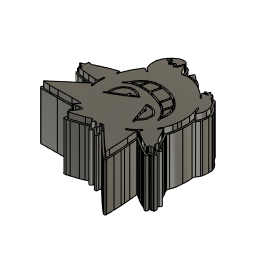
knop v2 (Autodesk Fusion 360 design; units mm, degrees)
Autodesk Fusion 360 part; units mm, degrees
(part 1 of 2)
sketch "Sketch5" plane through (0, 0, 0) normal (0, 0, 1) x (1, 0, 0)
  circle A0 centre (0, 52) radius 3.075
  circle A1 centre (0, 52) radius 12.5
  dimension "d73" = 6.15
  dimension "d74" = 25
  constraint concentric A0 A1
  measures "d73" diameter of A0
  measures "d74" diameter of A1
extrude "Extrude25" add sketch "Sketch5" along normal blind 14
sketch "Sketch6" plane through (0, 0, 0) normal (0, 0, -1) x (1, 0, 0)
  circle A0 centre (0, -52) radius 3.075
  circle A1 centre (0, -52) radius 12.5
  line L0 (0, -52) -> (0, -50.375)
  line L1 (0, -50.375) -> (-5.7654, -50.375)
  line L2 (0, -50.375) -> (4.6477, -50.375)
  dimension "d77" = 1.625
  constraint coincident A0.centre A1.centre
  constraint vertical L0
  constraint perpendicular L0 L1
  constraint perpendicular L0 L2
  measures "d77" distance of A0.centre L0.end
extrude "Extrude26" add sketch "Sketch6" against normal blind 14 contours A0 L1 L2 picked at (-0.148, -49.4191)
extrude "Extrude27" cut sketch "Sketch6" against normal blind 4 contours A0 L1 L2 picked at (-0.148, -49.4191)
sketch "Sketch7" plane through (0, 0, 14) normal (0, 0, 1) x (-1, 0, 0)
  arc A0 (-2.6106, -50.375) -> (2.6106, -50.375) centre (0, -52) ccw
  line L0 (-2.6106, -50.375) -> (2.6106, -50.375)
  circle A1 centre (0, -52) radius 12.5
extrude "Extrude28" add sketch "Sketch7" against normal blind 2 contours A0 L0
sketch "Sketch8" plane through (0, 0, 14) normal (0, 0, 1) x (-1, 0, 0)
  circle A0 centre (0, -52) radius 12.5
  spline S0 degree 3 poles (-7.7296, -35.2384) (-7.7669, -35.285) (-7.7902, -35.4107) (-7.7855, -35.555) knots 0 0 0 0 1 1 1 1
  spline S1 degree 3 poles (-7.7855, -35.555) (-7.7808, -35.6854) (-7.7576, -36.5886) (-7.7296, -37.5616) knots 0 0 0 0 1 1 1 1
  spline S2 degree 3 poles (-7.7296, -37.5616) (-7.7017, -38.5347) (-7.6691, -39.4053) (-7.6551, -39.4937) knots 0 0 0 0 1 1 1 1
  spline S3 degree 3 poles (-7.6551, -39.4937) (-7.6412, -39.5868) (-7.5993, -40.0245) (-7.562, -40.4714) knots 0 0 0 0 1 1 1 1
  spline S4 degree 3 poles (-7.562, -40.4714) (-7.427, -42.1521) (-7.278, -43.7118) (-7.2268, -44.0098) knots 0 0 0 0 1 1 1 1
  line L0 (-7.2268, -44.0098) -> (-7.1989, -44.1681)
  line L1 (-7.1989, -44.1681) -> (-7.3805, -44.0284)
  spline S5 degree 3 poles (-7.3805, -44.0284) (-7.6505, -43.8189) (-7.9857, -43.6001) (-8.2371, -43.4744) knots 0 0 0 0 1 1 1 1
  spline S6 degree 3 poles (-8.2371, -43.4744) (-8.3582, -43.4138) (-8.5164, -43.3114) (-8.5909, -43.2509) knots 0 0 0 0 1 1 1 1
  spline S7 degree 3 poles (-8.5909, -43.2509) (-8.6654, -43.1904) (-8.8191, -43.0926) (-8.9355, -43.0321) knots 0 0 0 0 1 1 1 1
  spline S8 degree 3 poles (-8.9355, -43.0321) (-9.0472, -42.9762) (-9.1962, -42.8877) (-9.2614, -42.8412) knots 0 0 0 0 1 1 1 1
  spline S9 degree 3 poles (-9.2614, -42.8412) (-9.3964, -42.7388) (-9.713, -42.5665) (-10.0063, -42.4268) knots 0 0 0 0 1 1 1 1
  spline S10 degree 3 poles (-10.0063, -42.4268) (-10.1227, -42.3756) (-10.2856, -42.2965) (-10.3694, -42.2546) knots 0 0 0 0 1 1 1 1
  spline S11 degree 3 poles (-10.3694, -42.2546) (-10.4579, -42.208) (-10.5556, -42.1708) (-10.5929, -42.1661) knots 0 0 0 0 1 1 1 1
  spline S12 degree 3 poles (-10.5929, -42.1661) (-10.6301, -42.1614) (-10.7279, -42.1149) (-10.8117, -42.059) knots 0 0 0 0 1 1 1 1
  spline S13 degree 3 poles (-10.8117, -42.059) (-10.8909, -42.0078) (-11.0398, -41.9194) (-11.1423, -41.8681) knots 0 0 0 0 1 1 1 1
  spline S14 degree 3 poles (-11.1423, -41.8681) (-11.24, -41.8123) (-11.403, -41.7052) (-11.5054, -41.6307) knots 0 0 0 0 1 1 1 1
  spline S15 degree 3 poles (-11.5054, -41.6307) (-11.7242, -41.4724) (-11.971, -41.4165) (-12.1246, -41.4864) knots 0 0 0 0 1 1 1 1
  spline S16 degree 3 poles (-12.1246, -41.4864) (-12.2689, -41.5515) (-12.3108, -41.7704) (-12.2457, -42.1242) knots 0 0 0 0 1 1 1 1
  spline S17 degree 3 poles (-12.2457, -42.1242) (-12.2177, -42.2732) (-12.1991, -42.4035) (-12.2084, -42.4082) knots 0 0 0 0 1 1 1 1
  spline S18 degree 3 poles (-12.2084, -42.4082) (-12.2177, -42.4175) (-12.2969, -42.4035) (-12.39, -42.3803) knots 0 0 0 0 1 1 1 1
  spline S19 degree 3 poles (-12.39, -42.3803) (-12.511, -42.343) (-12.6042, -42.3523) (-12.7531, -42.4035) knots 0 0 0 0 1 1 1 1
  spline S20 degree 3 poles (-12.7531, -42.4035) (-12.8602, -42.4408) (-13.0232, -42.4734) (-13.107, -42.4734) knots 0 0 0 0 1 1 1 1
  line L2 (-13.107, -42.4734) -> (-13.2653, -42.4734)
  line L3 (-13.2653, -42.4734) -> (-13.2653, -42.8924)
  line L4 (-13.2653, -42.8924) -> (-13.2653, -43.3067)
  line L5 (-13.2653, -43.3067) -> (-13.107, -43.4138)
  spline S21 degree 3 poles (-13.107, -43.4138) (-12.8975, -43.5582) (-12.5669, -43.8608) (-12.5669, -43.9073) knots 0 0 0 0 1 1 1 1
  spline S22 degree 3 poles (-12.5669, -43.9073) (-12.5669, -43.9306) (-12.6926, -44.0563) (-12.8462, -44.1913) knots 0 0 0 0 1 1 1 1
  spline S23 degree 3 poles (-12.8462, -44.1913) (-13.1302, -44.4381) (-13.2047, -44.5778) (-13.1489, -44.7547) knots 0 0 0 0 1 1 1 1
  spline S24 degree 3 poles (-13.1489, -44.7547) (-13.1209, -44.8478) (-12.9906, -44.9176) (-12.2503, -45.2482) knots 0 0 0 0 1 1 1 1
  spline S25 degree 3 poles (-12.2503, -45.2482) (-12.0827, -45.3227) (-11.9803, -45.4018) (-11.9244, -45.5042) knots 0 0 0 0 1 1 1 1
  spline S26 degree 3 poles (-11.9244, -45.5042) (-11.8825, -45.588) (-11.7894, -45.7231) (-11.7149, -45.8022) knots 0 0 0 0 1 1 1 1
  spline S27 degree 3 poles (-11.7149, -45.8022) (-11.6451, -45.886) (-11.5892, -45.9698) (-11.5892, -45.9838) knots 0 0 0 0 1 1 1 1
  spline S28 degree 3 poles (-11.5892, -45.9838) (-11.5892, -46.0024) (-11.4495, -46.3004) (-11.2819, -46.6542) knots 0 0 0 0 1 1 1 1
  spline S29 degree 3 poles (-11.2819, -46.6542) (-11.1143, -47.0034) (-10.956, -47.3339) (-10.9328, -47.3851) knots 0 0 0 0 1 1 1 1
  spline S30 degree 3 poles (-10.9328, -47.3851) (-10.9095, -47.4364) (-10.849, -47.5388) (-10.7977, -47.6179) knots 0 0 0 0 1 1 1 1
  spline S31 degree 3 poles (-10.7977, -47.6179) (-10.7465, -47.6924) (-10.6627, -47.8461) (-10.6115, -47.9531) knots 0 0 0 0 1 1 1 1
  spline S32 degree 3 poles (-10.6115, -47.9531) (-10.5556, -48.0602) (-10.4812, -48.158) (-10.4439, -48.172) knots 0 0 0 0 1 1 1 1
  spline S33 degree 3 poles (-10.4439, -48.172) (-10.4067, -48.1859) (-10.3787, -48.2278) (-10.3787, -48.2651) knots 0 0 0 0 1 1 1 1
  spline S34 degree 3 poles (-10.3787, -48.2651) (-10.3787, -48.3023) (-10.3135, -48.4466) (-10.2344, -48.5817) knots 0 0 0 0 1 1 1 1
  spline S35 degree 3 poles (-10.2344, -48.5817) (-10.1553, -48.7167) (-10.0808, -48.8657) (-10.0715, -48.9215) knots 0 0 0 0 1 1 1 1
  spline S36 degree 3 poles (-10.0715, -48.9215) (-10.0621, -48.9727) (-10.1366, -49.266) (-10.2391, -49.5733) knots 0 0 0 0 1 1 1 1
  spline S37 degree 3 poles (-10.2391, -49.5733) (-10.6208, -50.7373) (-10.6534, -50.9142) (-10.7698, -52.4878) knots 0 0 0 0 1 1 1 1
  spline S38 degree 3 poles (-10.7698, -52.4878) (-10.8396, -53.4515) (-10.8117, -54.7132) (-10.7093, -54.96) knots 0 0 0 0 1 1 1 1
  spline S39 degree 3 poles (-10.7093, -54.96) (-10.6348, -55.1509) (-10.6907, -55.3604) (-10.9141, -55.6956) knots 0 0 0 0 1 1 1 1
  spline S40 degree 3 poles (-10.9141, -55.6956) (-11.24, -56.1937) (-11.2819, -56.2682) (-11.389, -56.5336) knots 0 0 0 0 1 1 1 1
  spline S41 degree 3 poles (-11.389, -56.5336) (-11.5939, -57.0224) (-11.6544, -57.4228) (-11.6544, -58.3726) knots 0 0 0 0 1 1 1 1
  line L6 (-11.6544, -58.3726) -> (-11.6544, -59.2572)
  line L7 (-11.6544, -59.2572) -> (-11.4682, -59.6995)
  spline S42 degree 3 poles (-11.4682, -59.6995) (-11.3657, -59.9416) (-11.1795, -60.2814) (-11.0585, -60.4537) knots 0 0 0 0 1 1 1 1
  spline S43 degree 3 poles (-11.0585, -60.4537) (-10.8396, -60.7656) (-10.2251, -61.3755) (-10.132, -61.3755) knots 0 0 0 0 1 1 1 1
  spline S44 degree 3 poles (-10.132, -61.3755) (-10.104, -61.3755) (-9.969, -61.4407) (-9.834, -61.5245) knots 0 0 0 0 1 1 1 1
  spline S45 degree 3 poles (-9.834, -61.5245) (-9.6478, -61.6363) (-9.5733, -61.7154) (-9.536, -61.8411) knots 0 0 0 0 1 1 1 1
  spline S46 degree 3 poles (-9.536, -61.8411) (-9.5081, -61.9296) (-9.401, -62.1251) (-9.3033, -62.2787) knots 0 0 0 0 1 1 1 1
  spline S47 degree 3 poles (-9.3033, -62.2787) (-9.2008, -62.4277) (-9.1217, -62.5674) (-9.1217, -62.586) knots 0 0 0 0 1 1 1 1
  spline S48 degree 3 poles (-9.1217, -62.586) (-9.1217, -62.6046) (-9.0193, -62.7164) (-8.8889, -62.8374) knots 0 0 0 0 1 1 1 1
  spline S49 degree 3 poles (-8.8889, -62.8374) (-8.6096, -63.0981) (-8.4606, -63.1168) (-8.3349, -62.9073) knots 0 0 0 0 1 1 1 1
  line L8 (-8.3349, -62.9073) -> (-8.2418, -62.7583)
  line L9 (-8.2418, -62.7583) -> (-8.144, -62.9724)
  spline S50 degree 3 poles (-8.144, -62.9724) (-8.0648, -63.1447) (-8.0043, -63.2006) (-7.8181, -63.2797) knots 0 0 0 0 1 1 1 1
  spline S51 degree 3 poles (-7.8181, -63.2797) (-7.4084, -63.4566) (-7.3292, -63.4101) (-7.2548, -62.9538) knots 0 0 0 0 1 1 1 1
  spline S52 degree 3 poles (-7.2548, -62.9538) (-7.2268, -62.7909) (-7.1989, -62.6512) (-7.1942, -62.6465) knots 0 0 0 0 1 1 1 1
  spline S53 degree 3 poles (-7.1942, -62.6465) (-7.1849, -62.6372) (-7.0871, -62.6838) (-6.9754, -62.749) knots 0 0 0 0 1 1 1 1
  spline S54 degree 3 poles (-6.9754, -62.749) (-6.8637, -62.8095) (-6.7147, -62.8654) (-6.6449, -62.8654) knots 0 0 0 0 1 1 1 1
  spline S55 degree 3 poles (-6.6449, -62.8654) (-6.3981, -62.8654) (-6.3003, -62.5395) (-6.4447, -62.1996) knots 0 0 0 0 1 1 1 1
  spline S56 degree 3 poles (-6.4447, -62.1996) (-6.5238, -62.0041) (-6.5378, -61.748) (-6.4633, -61.748) knots 0 0 0 0 1 1 1 1
  spline S57 degree 3 poles (-6.4633, -61.748) (-6.4353, -61.748) (-6.3562, -61.8085) (-6.2864, -61.8783) knots 0 0 0 0 1 1 1 1
  spline S58 degree 3 poles (-6.2864, -61.8783) (-6.1141, -62.046) (-5.467, -62.4789) (-5.0247, -62.7164) knots 0 0 0 0 1 1 1 1
  spline S59 degree 3 poles (-5.0247, -62.7164) (-4.5032, -62.9957) (-4.4194, -63.033) (-4.1261, -63.1633) knots 0 0 0 0 1 1 1 1
  spline S60 degree 3 poles (-4.1261, -63.1633) (-3.9352, -63.2518) (-3.8282, -63.3309) (-3.763, -63.4473) knots 0 0 0 0 1 1 1 1
  spline S61 degree 3 poles (-3.763, -63.4473) (-3.7071, -63.5358) (-3.6512, -63.6103) (-3.6326, -63.6103) knots 0 0 0 0 1 1 1 1
  spline S62 degree 3 poles (-3.6326, -63.6103) (-3.614, -63.6103) (-3.5674, -63.6661) (-3.5302, -63.736) knots 0 0 0 0 1 1 1 1
  spline S63 degree 3 poles (-3.5302, -63.736) (-3.4929, -63.8058) (-3.3719, -63.9455) (-3.2648, -64.0479) knots 0 0 0 0 1 1 1 1
  spline S64 degree 3 poles (-3.2648, -64.0479) (-3.1531, -64.155) (-2.9762, -64.3226) (-2.8691, -64.4297) knots 0 0 0 0 1 1 1 1
  spline S65 degree 3 poles (-2.8691, -64.4297) (-2.2918, -64.9884) (-1.4631, -65.3143) (-1.2442, -65.0628) knots 0 0 0 0 1 1 1 1
  spline S66 degree 3 poles (-1.2442, -65.0628) (-1.2023, -65.0209) (-1.0953, -64.7835) (-0.9975, -64.5414) knots 0 0 0 0 1 1 1 1
  spline S67 degree 3 poles (-0.9975, -64.5414) (-0.6716, -63.7127) (-0.6157, -63.6429) (-0.2014, -63.5916) knots 0 0 0 0 1 1 1 1
  spline S68 degree 3 poles (-0.2014, -63.5916) (0.0314, -63.5637) (0.0407, -63.5637) (0.1851, -63.736) knots 0 0 0 0 1 1 1 1
  spline S69 degree 3 poles (0.1851, -63.736) (0.2642, -63.8337) (0.3899, -63.9734) (0.4644, -64.0526) knots 0 0 0 0 1 1 1 1
  spline S70 degree 3 poles (0.4644, -64.0526) (0.5901, -64.1783) (1.1302, -65.2724) (1.2885, -65.724) knots 0 0 0 0 1 1 1 1
  spline S71 degree 3 poles (1.2885, -65.724) (1.4654, -66.2175) (1.7866, -66.5853) (2.1405, -66.711) knots 0 0 0 0 1 1 1 1
  spline S72 degree 3 poles (2.1405, -66.711) (2.2475, -66.7482) (2.6107, -66.7715) (3.1368, -66.7761) knots 0 0 0 0 1 1 1 1
  spline S73 degree 3 poles (3.1368, -66.7761) (3.9562, -66.7808) (3.9655, -66.7761) (4.1843, -66.6504) knots 0 0 0 0 1 1 1 1
  spline S74 degree 3 poles (4.1843, -66.6504) (4.3054, -66.5806) (4.4264, -66.5015) (4.4543, -66.4735) knots 0 0 0 0 1 1 1 1
  spline S75 degree 3 poles (4.4543, -66.4735) (4.4823, -66.4502) (4.6313, -66.3432) (4.7802, -66.2407) knots 0 0 0 0 1 1 1 1
  spline S76 degree 3 poles (4.7802, -66.2407) (5.3529, -65.8497) (6.1863, -64.872) (6.5029, -64.2155) knots 0 0 0 0 1 1 1 1
  spline S77 degree 3 poles (6.5029, -64.2155) (6.596, -64.0246) (6.6891, -63.8291) (6.7077, -63.7872) knots 0 0 0 0 1 1 1 1
  spline S78 degree 3 poles (6.7077, -63.7872) (6.866, -63.4892) (7.0615, -62.2089) (7.0196, -61.7806) knots 0 0 0 0 1 1 1 1
  spline S79 degree 3 poles (7.0196, -61.7806) (6.9498, -61.0962) (6.8753, -60.6725) (6.7729, -60.4258) knots 0 0 0 0 1 1 1 1
  spline S80 degree 3 poles (6.7729, -60.4258) (6.6332, -60.0812) (6.6332, -60.0673) (6.7775, -59.9323) knots 0 0 0 0 1 1 1 1
  spline S81 degree 3 poles (6.7775, -59.9323) (6.8427, -59.8717) (6.8939, -59.7972) (6.8939, -59.7647) knots 0 0 0 0 1 1 1 1
  spline S82 degree 3 poles (6.8939, -59.7647) (6.8939, -59.7321) (6.9219, -59.6762) (6.9591, -59.639) knots 0 0 0 0 1 1 1 1
  spline S83 degree 3 poles (6.9591, -59.639) (7.1593, -59.4434) (8.4303, -57.1575) (8.4303, -57.0038) knots 0 0 0 0 1 1 1 1
  spline S84 degree 3 poles (8.4303, -57.0038) (8.4303, -56.9759) (8.4955, -56.8316) (8.57, -56.6872) knots 0 0 0 0 1 1 1 1
  spline S85 degree 3 poles (8.57, -56.6872) (8.6491, -56.5429) (8.7097, -56.4032) (8.7097, -56.3707) knots 0 0 0 0 1 1 1 1
  spline S86 degree 3 poles (8.7097, -56.3707) (8.7097, -56.2636) (8.8726, -56.1705) (9.2683, -56.0494) knots 0 0 0 0 1 1 1 1
  spline S87 degree 3 poles (9.2683, -56.0494) (10.1064, -55.798) (10.5161, -55.6537) (10.7489, -55.5373) knots 0 0 0 0 1 1 1 1
  spline S88 degree 3 poles (10.7489, -55.5373) (10.8792, -55.4721) (11.0328, -55.4162) (11.0841, -55.4162) knots 0 0 0 0 1 1 1 1
  spline S89 degree 3 poles (11.0841, -55.4162) (11.1353, -55.4162) (11.3913, -55.3138) (11.6567, -55.1881) knots 0 0 0 0 1 1 1 1
  spline S90 degree 3 poles (11.6567, -55.1881) (11.9174, -55.0624) (12.1828, -54.946) (12.248, -54.9274) knots 0 0 0 0 1 1 1 1
  spline S91 degree 3 poles (12.248, -54.9274) (12.3132, -54.9088) (12.4482, -54.8436) (12.5506, -54.7877) knots 0 0 0 0 1 1 1 1
  spline S92 degree 3 poles (12.5506, -54.7877) (12.653, -54.7272) (12.8486, -54.648) (12.9789, -54.6015) knots 0 0 0 0 1 1 1 1
  spline S93 degree 3 poles (12.9789, -54.6015) (13.1139, -54.5596) (13.235, -54.5084) (13.249, -54.4851) knots 0 0 0 0 1 1 1 1
  spline S94 degree 3 poles (13.249, -54.4851) (13.2955, -54.4106) (14.2639, -53.9683) (14.3384, -53.9869) knots 0 0 0 0 1 1 1 1
  spline S95 degree 3 poles (14.3384, -53.9869) (14.3803, -54.0009) (14.5619, -54.0614) (14.7388, -54.1266) knots 0 0 0 0 1 1 1 1
  spline S96 degree 3 poles (14.7388, -54.1266) (15.0833, -54.2523) (15.2882, -54.2477) (15.3487, -54.1173) knots 0 0 0 0 1 1 1 1
  spline S97 degree 3 poles (15.3487, -54.1173) (15.372, -54.0754) (15.3999, -53.8333) (15.4139, -53.5772) knots 0 0 0 0 1 1 1 1
  line L10 (15.4139, -53.5772) -> (15.4371, -53.1117)
  line L11 (15.4371, -53.1117) -> (15.7863, -52.9953)
  spline S98 degree 3 poles (15.7863, -52.9953) (16.3869, -52.7951) (16.6756, -52.5716) (16.6057, -52.3621) knots 0 0 0 0 1 1 1 1
  spline S99 degree 3 poles (16.6057, -52.3621) (16.5731, -52.2597) (16.0796, -51.9291) (15.8329, -51.8407) knots 0 0 0 0 1 1 1 1
  spline S100 degree 3 poles (15.8329, -51.8407) (15.7444, -51.8081) (15.6373, -51.7708) (15.6001, -51.7569) knots 0 0 0 0 1 1 1 1
  spline S101 degree 3 poles (15.6001, -51.7569) (15.5535, -51.7382) (15.6001, -51.6917) (15.7491, -51.6172) knots 0 0 0 0 1 1 1 1
  spline S102 degree 3 poles (15.7491, -51.6172) (15.9353, -51.5241) (15.9726, -51.4822) (15.9726, -51.3704) knots 0 0 0 0 1 1 1 1
  spline S103 degree 3 poles (15.9726, -51.3704) (15.9726, -51.147) (15.8143, -51.0632) (14.9809, -50.849) knots 0 0 0 0 1 1 1 1
  spline S104 degree 3 poles (14.9809, -50.849) (14.7202, -50.7838) (13.7937, -50.6674) (13.519, -50.6674) knots 0 0 0 0 1 1 1 1
  spline S105 degree 3 poles (13.519, -50.6674) (13.3886, -50.6674) (13.2629, -50.6441) (13.249, -50.6209) knots 0 0 0 0 1 1 1 1
  spline S106 degree 3 poles (13.249, -50.6209) (13.235, -50.5929) (13.0162, -50.5743) (12.7555, -50.5743) knots 0 0 0 0 1 1 1 1
  spline S107 degree 3 poles (12.7555, -50.5743) (12.4994, -50.5743) (12.1363, -50.5417) (11.9454, -50.5045) knots 0 0 0 0 1 1 1 1
  spline S108 degree 3 poles (11.9454, -50.5045) (11.7545, -50.4626) (11.3215, -50.4114) (10.9816, -50.3881) knots 0 0 0 0 1 1 1 1
  spline S109 degree 3 poles (10.9816, -50.3881) (10.2786, -50.3369) (9.8829, -50.2763) (9.8084, -50.2018) knots 0 0 0 0 1 1 1 1
  spline S110 degree 3 poles (9.8084, -50.2018) (9.7572, -50.146) (9.962, -49.9411) (10.5906, -49.4104) knots 0 0 0 0 1 1 1 1
  spline S111 degree 3 poles (10.5906, -49.4104) (10.7582, -49.2707) (11.0282, -49.0333) (11.1865, -48.8843) knots 0 0 0 0 1 1 1 1
  spline S112 degree 3 poles (11.1865, -48.8843) (11.3448, -48.74) (11.4891, -48.6189) (11.5031, -48.6189) knots 0 0 0 0 1 1 1 1
  spline S113 degree 3 poles (11.5031, -48.6189) (11.5217, -48.6189) (11.6055, -48.5537) (11.694, -48.4792) knots 0 0 0 0 1 1 1 1
  spline S114 degree 3 poles (11.694, -48.4792) (11.7824, -48.4001) (11.9267, -48.2744) (12.0152, -48.1999) knots 0 0 0 0 1 1 1 1
  spline S115 degree 3 poles (12.0152, -48.1999) (12.1037, -48.1207) (12.3364, -47.9206) (12.5273, -47.7529) knots 0 0 0 0 1 1 1 1
  spline S116 degree 3 poles (12.5273, -47.7529) (12.7182, -47.5807) (12.937, -47.3991) (13.0208, -47.3432) knots 0 0 0 0 1 1 1 1
  spline S117 degree 3 poles (13.0208, -47.3432) (13.1745, -47.2408) (14.2127, -46.3749) (14.4594, -46.1374) knots 0 0 0 0 1 1 1 1
  spline S118 degree 3 poles (14.4594, -46.1374) (14.5386, -46.0676) (14.6643, -45.9465) (14.7388, -45.8767) knots 0 0 0 0 1 1 1 1
  spline S119 degree 3 poles (14.7388, -45.8767) (14.8179, -45.8022) (15.1531, -45.5089) (15.4837, -45.2202) knots 0 0 0 0 1 1 1 1
  spline S120 degree 3 poles (15.4837, -45.2202) (15.8189, -44.9362) (16.1774, -44.6197) (16.2845, -44.5219) knots 0 0 0 0 1 1 1 1
  spline S121 degree 3 poles (16.2845, -44.5219) (16.3916, -44.4241) (16.5685, -44.2798) (16.6802, -44.2053) knots 0 0 0 0 1 1 1 1
  spline S122 degree 3 poles (16.6802, -44.2053) (16.792, -44.1308) (16.9177, -44.0284) (16.9596, -43.9772) knots 0 0 0 0 1 1 1 1
  spline S123 degree 3 poles (16.9596, -43.9772) (17.0992, -43.8235) (17.2808, -43.4464) (17.2529, -43.3626) knots 0 0 0 0 1 1 1 1
  spline S124 degree 3 poles (17.2529, -43.3626) (17.2389, -43.3207) (17.1504, -43.2369) (17.0573, -43.1717) knots 0 0 0 0 1 1 1 1
  line L12 (17.0573, -43.1717) -> (16.8851, -43.0553)
  line L13 (16.8851, -43.0553) -> (12.5785, -43.06)
  spline S125 degree 3 poles (12.5785, -43.06) (9.0262, -43.0693) (8.1975, -43.0786) (7.8623, -43.1391) knots 0 0 0 0 1 1 1 1
  spline S126 degree 3 poles (7.8623, -43.1391) (7.4666, -43.2043) (7.3409, -43.1764) (7.5597, -43.074) knots 0 0 0 0 1 1 1 1
  spline S127 degree 3 poles (7.5597, -43.074) (7.6156, -43.046) (7.7133, -42.9529) (7.7785, -42.8691) knots 0 0 0 0 1 1 1 1
  spline S128 degree 3 poles (7.7785, -42.8691) (7.8437, -42.7853) (7.9927, -42.5851) (8.1184, -42.4268) knots 0 0 0 0 1 1 1 1
  spline S129 degree 3 poles (8.1184, -42.4268) (8.3512, -42.1195) (8.3977, -41.9287) (8.2627, -41.8169) knots 0 0 0 0 1 1 1 1
  spline S130 degree 3 poles (8.2627, -41.8169) (8.2022, -41.7657) (8.0951, -41.7704) (7.6249, -41.8355) knots 0 0 0 0 1 1 1 1
  spline S131 degree 3 poles (7.6249, -41.8355) (7.3129, -41.8821) (6.9545, -41.9147) (6.8241, -41.9147) knots 0 0 0 0 1 1 1 1
  spline S132 degree 3 poles (6.8241, -41.9147) (6.6984, -41.9147) (6.4284, -41.9566) (6.2282, -42.0032) knots 0 0 0 0 1 1 1 1
  line L14 (6.2282, -42.0032) -> (5.865, -42.087)
  line L15 (5.865, -42.087) -> (5.9395, -41.9892)
  spline S133 degree 3 poles (5.9395, -41.9892) (5.9814, -41.938) (6.0559, -41.803) (6.1071, -41.6959) knots 0 0 0 0 1 1 1 1
  spline S134 degree 3 poles (6.1071, -41.6959) (6.1583, -41.5888) (6.2142, -41.4864) (6.2375, -41.4771) knots 0 0 0 0 1 1 1 1
  spline S135 degree 3 poles (6.2375, -41.4771) (6.3027, -41.4352) (6.6611, -40.8113) (6.9731, -40.1967) knots 0 0 0 0 1 1 1 1
  spline S136 degree 3 poles (6.9731, -40.1967) (7.3502, -39.4518) (7.3595, -39.2749) (7.0103, -39.2423) knots 0 0 0 0 1 1 1 1
  spline S137 degree 3 poles (7.0103, -39.2423) (6.9079, -39.233) (6.6891, -39.2656) (6.5215, -39.3122) knots 0 0 0 0 1 1 1 1
  spline S138 degree 3 poles (6.5215, -39.3122) (6.3539, -39.3634) (6, -39.4611) (5.73, -39.5356) knots 0 0 0 0 1 1 1 1
  spline S139 degree 3 poles (5.73, -39.5356) (4.8501, -39.7824) (3.2485, -40.3318) (2.8202, -40.5413) knots 0 0 0 0 1 1 1 1
  spline S140 degree 3 poles (2.8202, -40.5413) (2.2382, -40.8253) (1.9542, -40.9417) (1.9123, -40.9137) knots 0 0 0 0 1 1 1 1
  spline S141 degree 3 poles (1.9123, -40.9137) (1.889, -40.8998) (1.8146, -40.774) (1.7494, -40.6297) knots 0 0 0 0 1 1 1 1
  spline S142 degree 3 poles (1.7494, -40.6297) (1.6842, -40.49) (1.5538, -40.2899) (1.4607, -40.1874) knots 0 0 0 0 1 1 1 1
  spline S143 degree 3 poles (1.4607, -40.1874) (1.1767, -39.8755) (0.9858, -39.95) (0.7018, -40.504) knots 0 0 0 0 1 1 1 1
  spline S144 degree 3 poles (0.7018, -40.504) (0.646, -40.6158) (0.5901, -40.7042) (0.5761, -40.7042) knots 0 0 0 0 1 1 1 1
  spline S145 degree 3 poles (0.5761, -40.7042) (0.5668, -40.7042) (0.4877, -40.6344) (0.4039, -40.5506) knots 0 0 0 0 1 1 1 1
  spline S146 degree 3 poles (0.4039, -40.5506) (0.3201, -40.4714) (0.1199, -40.2759) (-0.0477, -40.1176) knots 0 0 0 0 1 1 1 1
  spline S147 degree 3 poles (-0.0477, -40.1176) (-0.2107, -39.964) (-0.4341, -39.7405) (-0.5412, -39.6194) knots 0 0 0 0 1 1 1 1
  spline S148 degree 3 poles (-0.5412, -39.6194) (-0.6483, -39.503) (-0.7833, -39.4006) (-0.8438, -39.3913) knots 0 0 0 0 1 1 1 1
  spline S149 degree 3 poles (-0.8438, -39.3913) (-1.0534, -39.3634) (-1.1139, -39.4844) (-1.1884, -40.1036) knots 0 0 0 0 1 1 1 1
  spline S150 degree 3 poles (-1.1884, -40.1036) (-1.2722, -40.802) (-1.2861, -40.8579) (-1.3606, -40.7182) knots 0 0 0 0 1 1 1 1
  spline S151 degree 3 poles (-1.3606, -40.7182) (-1.3932, -40.6623) (-1.5422, -40.5087) (-1.6912, -40.369) knots 0 0 0 0 1 1 1 1
  spline S152 degree 3 poles (-1.6912, -40.369) (-1.8448, -40.234) (-2.0124, -40.071) (-2.0636, -40.0105) knots 0 0 0 0 1 1 1 1
  spline S153 degree 3 poles (-2.0636, -40.0105) (-2.1195, -39.9453) (-2.194, -39.8615) (-2.2406, -39.8243) knots 0 0 0 0 1 1 1 1
  spline S154 degree 3 poles (-2.2406, -39.8243) (-2.2825, -39.7824) (-2.5339, -39.5403) (-2.7992, -39.2842) knots 0 0 0 0 1 1 1 1
  spline S155 degree 3 poles (-2.7992, -39.2842) (-3.3766, -38.7255) (-4.2658, -37.8968) (-5.0945, -37.1333) knots 0 0 0 0 1 1 1 1
  spline S156 degree 3 poles (-5.0945, -37.1333) (-5.4251, -36.8307) (-5.7789, -36.5048) (-5.872, -36.4163) knots 0 0 0 0 1 1 1 1
  spline S157 degree 3 poles (-5.872, -36.4163) (-6.1746, -36.137) (-6.4726, -35.8902) (-6.6774, -35.7459) knots 0 0 0 0 1 1 1 1
  spline S158 degree 3 poles (-6.6774, -35.7459) (-6.7845, -35.6667) (-7.008, -35.5084) (-7.1663, -35.3827) knots 0 0 0 0 1 1 1 1
  spline S159 degree 3 poles (-7.1663, -35.3827) (-7.4689, -35.1546) (-7.6226, -35.1127) (-7.7296, -35.2384) knots 0 0 0 0 1 1 1 1
  spline S160 degree 3 poles (-7.3153, -35.6807) (-7.3479, -35.6993) (-7.3618, -35.7273) (-7.3525, -35.7366) knots 0 0 0 0 1 1 1 1
  spline S161 degree 3 poles (-7.3525, -35.7366) (-7.3386, -35.7459) (-7.1523, -35.8995) (-6.9335, -36.0764) knots 0 0 0 0 1 1 1 1
  spline S162 degree 3 poles (-6.9335, -36.0764) (-6.5704, -36.3698) (-5.5275, -37.2962) (-5.4204, -37.4173) knots 0 0 0 0 1 1 1 1
  spline S163 degree 3 poles (-5.4204, -37.4173) (-5.3925, -37.4499) (-4.9735, -37.8363) (-4.4893, -38.2832) knots 0 0 0 0 1 1 1 1
  spline S164 degree 3 poles (-4.4893, -38.2832) (-3.6, -39.098) (-2.9715, -39.6939) (-2.4454, -40.22) knots 0 0 0 0 1 1 1 1
  spline S165 degree 3 poles (-2.4454, -40.22) (-2.2871, -40.3783) (-2.0031, -40.6483) (-1.8122, -40.8206) knots 0 0 0 0 1 1 1 1
  spline S166 degree 3 poles (-1.8122, -40.8206) (-1.6214, -40.9929) (-1.3979, -41.1931) (-1.3187, -41.2629) knots 0 0 0 0 1 1 1 1
  spline S167 degree 3 poles (-1.3187, -41.2629) (-1.0813, -41.4724) (-0.9835, -41.5096) (-0.7135, -41.4771) knots 0 0 0 0 1 1 1 1
  spline S168 degree 3 poles (-0.7135, -41.4771) (-0.369, -41.4352) (-0.2293, -41.3746) (-0.2293, -41.2629) knots 0 0 0 0 1 1 1 1
  spline S169 degree 3 poles (-0.2293, -41.2629) (-0.2293, -41.1465) (-0.3969, -41.0999) (-0.6809, -41.1418) knots 0 0 0 0 1 1 1 1
  line L16 (-0.6809, -41.1418) -> (-0.8951, -41.1698)
  line L17 (-0.8951, -41.1698) -> (-0.8671, -40.6949)
  spline S170 degree 3 poles (-0.8671, -40.6949) (-0.8392, -40.2014) (-0.8066, -40.0384) (-0.7368, -40.0617) knots 0 0 0 0 1 1 1 1
  spline S171 degree 3 poles (-0.7368, -40.0617) (-0.7181, -40.071) (-0.504, -40.2666) (-0.2665, -40.4994) knots 0 0 0 0 1 1 1 1
  spline S172 degree 3 poles (-0.2665, -40.4994) (0.4132, -41.1605) (0.8555, -41.4445) (0.9067, -41.2489) knots 0 0 0 0 1 1 1 1
  spline S173 degree 3 poles (0.9067, -41.2489) (0.9719, -40.9929) (1.1488, -40.518) (1.1767, -40.518) knots 0 0 0 0 1 1 1 1
  spline S174 degree 3 poles (1.1767, -40.518) (1.1953, -40.518) (1.2978, -40.6902) (1.4049, -40.8998) knots 0 0 0 0 1 1 1 1
  spline S175 degree 3 poles (1.4049, -40.8998) (1.647, -41.3933) (1.6656, -41.4165) (1.8378, -41.3886) knots 0 0 0 0 1 1 1 1
  spline S176 degree 3 poles (1.8378, -41.3886) (1.9868, -41.3653) (2.7178, -41.0767) (3.053, -40.9044) knots 0 0 0 0 1 1 1 1
  spline S177 degree 3 poles (3.053, -40.9044) (3.3696, -40.7461) (5.1667, -40.1548) (6.3818, -39.815) knots 0 0 0 0 1 1 1 1
  spline S178 degree 3 poles (6.3818, -39.815) (6.7589, -39.7079) (6.7868, -39.7079) (6.6984, -39.8057) knots 0 0 0 0 1 1 1 1
  spline S179 degree 3 poles (6.6984, -39.8057) (6.6565, -39.8522) (6.6099, -39.936) (6.596, -39.9919) knots 0 0 0 0 1 1 1 1
  spline S180 degree 3 poles (6.596, -39.9919) (6.5634, -40.0897) (5.9861, -41.0906) (5.6695, -41.5888) knots 0 0 0 0 1 1 1 1
  spline S181 degree 3 poles (5.6695, -41.5888) (5.4786, -41.8914) (5.2831, -42.3663) (5.325, -42.4129) knots 0 0 0 0 1 1 1 1
  spline S182 degree 3 poles (5.325, -42.4129) (5.3855, -42.4734) (5.8883, -42.4827) (6.2654, -42.4268) knots 0 0 0 0 1 1 1 1
  spline S183 degree 3 poles (6.2654, -42.4268) (6.4703, -42.3989) (6.8055, -42.357) (7.0103, -42.3337) knots 0 0 0 0 1 1 1 1
  spline S184 degree 3 poles (7.0103, -42.3337) (7.2152, -42.3104) (7.4666, -42.2778) (7.569, -42.2639) knots 0 0 0 0 1 1 1 1
  line L18 (7.569, -42.2639) -> (7.7552, -42.2359)
  line L19 (7.7552, -42.2359) -> (7.6342, -42.343)
  spline S185 degree 3 poles (7.6342, -42.343) (7.5085, -42.4548) (7.1267, -42.9576) (7.1267, -43.0134) knots 0 0 0 0 1 1 1 1
  spline S186 degree 3 poles (7.1267, -43.0134) (7.1267, -43.0833) (6.9684, -43.2183) (6.8846, -43.2183) knots 0 0 0 0 1 1 1 1
  spline S187 degree 3 poles (6.8846, -43.2183) (6.7682, -43.2183) (6.7263, -43.3487) (6.8101, -43.4371) knots 0 0 0 0 1 1 1 1
  spline S188 degree 3 poles (6.8101, -43.4371) (6.8707, -43.4976) (7.1919, -43.5069) (9.1985, -43.5069) knots 0 0 0 0 1 1 1 1
  spline S189 degree 3 poles (9.1985, -43.5069) (10.4695, -43.5069) (12.0757, -43.479) (12.7648, -43.4464) knots 0 0 0 0 1 1 1 1
  spline S190 degree 3 poles (12.7648, -43.4464) (13.4585, -43.4185) (14.4362, -43.4045) (14.939, -43.4185) knots 0 0 0 0 1 1 1 1
  spline S191 degree 3 poles (14.939, -43.4185) (15.8422, -43.4418) (16.7175, -43.5302) (16.7175, -43.6001) knots 0 0 0 0 1 1 1 1
  spline S192 degree 3 poles (16.7175, -43.6001) (16.7175, -43.6187) (16.6616, -43.6699) (16.5918, -43.7165) knots 0 0 0 0 1 1 1 1
  spline S193 degree 3 poles (16.5918, -43.7165) (16.5173, -43.7584) (16.3916, -43.8654) (16.3078, -43.9492) knots 0 0 0 0 1 1 1 1
  spline S194 degree 3 poles (16.3078, -43.9492) (16.224, -44.033) (16.0051, -44.2239) (15.8189, -44.3682) knots 0 0 0 0 1 1 1 1
  spline S195 degree 3 poles (15.8189, -44.3682) (15.3906, -44.7128) (14.3431, -45.6299) (13.8309, -46.1048) knots 0 0 0 0 1 1 1 1
  spline S196 degree 3 poles (13.8309, -46.1048) (13.6121, -46.3097) (13.235, -46.6263) (12.9929, -46.8125) knots 0 0 0 0 1 1 1 1
  spline S197 degree 3 poles (12.9929, -46.8125) (12.7508, -46.9941) (12.2945, -47.3665) (11.9826, -47.6366) knots 0 0 0 0 1 1 1 1
  spline S198 degree 3 poles (11.9826, -47.6366) (11.666, -47.9066) (11.2424, -48.2651) (11.0328, -48.4327) knots 0 0 0 0 1 1 1 1
  spline S199 degree 3 poles (11.0328, -48.4327) (10.828, -48.6003) (10.5347, -48.8517) (10.3904, -48.9914) knots 0 0 0 0 1 1 1 1
  spline S200 degree 3 poles (10.3904, -48.9914) (9.9434, -49.415) (9.7293, -49.6059) (9.7153, -49.5919) knots 0 0 0 0 1 1 1 1
  spline S201 degree 3 poles (9.7153, -49.5919) (9.706, -49.5826) (9.6734, -49.4383) (9.6455, -49.2754) knots 0 0 0 0 1 1 1 1
  spline S202 degree 3 poles (9.6455, -49.2754) (9.557, -48.8144) (9.5197, -48.7493) (9.3708, -48.7679) knots 0 0 0 0 1 1 1 1
  spline S203 degree 3 poles (9.3708, -48.7679) (9.259, -48.7819) (9.2451, -48.8005) (9.2497, -48.9448) knots 0 0 0 0 1 1 1 1
  spline S204 degree 3 poles (9.2497, -48.9448) (9.2497, -49.0333) (9.2916, -49.2754) (9.3382, -49.4802) knots 0 0 0 0 1 1 1 1
  spline S205 degree 3 poles (9.3382, -49.4802) (9.4173, -49.8434) (9.4313, -50.3136) (9.3894, -52.0408) knots 0 0 0 0 1 1 1 1
  spline S206 degree 3 poles (9.3894, -52.0408) (9.3847, -52.2923) (9.394, -52.3202) (9.4825, -52.3342) knots 0 0 0 0 1 1 1 1
  spline S207 degree 3 poles (9.4825, -52.3342) (9.6268, -52.3528) (9.6455, -52.2643) (9.6874, -51.4682) knots 0 0 0 0 1 1 1 1
  spline S208 degree 3 poles (9.6874, -51.4682) (9.706, -51.0771) (9.7339, -50.7466) (9.7525, -50.7279) knots 0 0 0 0 1 1 1 1
  spline S209 degree 3 poles (9.7525, -50.7279) (9.7665, -50.7093) (10.0691, -50.7233) (10.423, -50.7512) knots 0 0 0 0 1 1 1 1
  spline S210 degree 3 poles (10.423, -50.7512) (10.7721, -50.7792) (11.5729, -50.849) (12.2014, -50.9002) knots 0 0 0 0 1 1 1 1
  spline S211 degree 3 poles (12.2014, -50.9002) (12.83, -50.9514) (13.5423, -51.0212) (13.7844, -51.0585) knots 0 0 0 0 1 1 1 1
  spline S212 degree 3 poles (13.7844, -51.0585) (14.9855, -51.2447) (15.209, -51.2866) (15.2928, -51.3285) knots 0 0 0 0 1 1 1 1
  spline S213 degree 3 poles (15.2928, -51.3285) (15.372, -51.3704) (15.372, -51.3797) (15.3068, -51.4496) knots 0 0 0 0 1 1 1 1
  spline S214 degree 3 poles (15.3068, -51.4496) (15.2416, -51.5101) (15.209, -51.5148) (15.0461, -51.4589) knots 0 0 0 0 1 1 1 1
  spline S215 degree 3 poles (15.0461, -51.4589) (14.9436, -51.4263) (14.8272, -51.4123) (14.79, -51.4263) knots 0 0 0 0 1 1 1 1
  spline S216 degree 3 poles (14.79, -51.4263) (14.7015, -51.4589) (14.6969, -51.5939) (14.776, -51.6917) knots 0 0 0 0 1 1 1 1
  spline S217 degree 3 poles (14.776, -51.6917) (14.8598, -51.7988) (15.4744, -52.1572) (15.5815, -52.1572) knots 0 0 0 0 1 1 1 1
  spline S218 degree 3 poles (15.5815, -52.1572) (15.628, -52.1619) (15.763, -52.2131) (15.8794, -52.2736) knots 0 0 0 0 1 1 1 1
  line L20 (15.8794, -52.2736) -> (16.0889, -52.3807)
  line L21 (16.0889, -52.3807) -> (15.9027, -52.4599)
  spline S219 degree 3 poles (15.9027, -52.4599) (15.0181, -52.8277) (14.9949, -52.8509) (14.9949, -53.3957) knots 0 0 0 0 1 1 1 1
  line L22 (14.9949, -53.3957) -> (14.9949, -53.7821)
  line L23 (14.9949, -53.7821) -> (14.7062, -53.661)
  spline S220 degree 3 poles (14.7062, -53.661) (14.3617, -53.5214) (14.1754, -53.5353) (13.7611, -53.7355) knots 0 0 0 0 1 1 1 1
  spline S221 degree 3 poles (13.7611, -53.7355) (13.6075, -53.81) (13.2629, -53.973) (12.9929, -54.094) knots 0 0 0 0 1 1 1 1
  spline S222 degree 3 poles (12.9929, -54.094) (12.7229, -54.2151) (12.234, -54.4339) (11.8988, -54.5875) knots 0 0 0 0 1 1 1 1
  spline S223 degree 3 poles (11.8988, -54.5875) (11.5683, -54.7412) (11.0841, -54.9414) (10.828, -55.0391) knots 0 0 0 0 1 1 1 1
  spline S224 degree 3 poles (10.828, -55.0391) (10.2786, -55.2486) (8.8912, -55.7049) (8.8679, -55.6816) knots 0 0 0 0 1 1 1 1
  spline S225 degree 3 poles (8.8679, -55.6816) (8.8586, -55.677) (8.8819, -55.5419) (8.9192, -55.393) knots 0 0 0 0 1 1 1 1
  spline S226 degree 3 poles (8.9192, -55.393) (8.9564, -55.2393) (8.9843, -55.0531) (8.989, -54.9833) knots 0 0 0 0 1 1 1 1
  spline S227 degree 3 poles (8.989, -54.9833) (8.989, -54.8389) (8.8819, -54.7737) (8.7841, -54.8575) knots 0 0 0 0 1 1 1 1
  spline S228 degree 3 poles (8.7841, -54.8575) (8.7143, -54.9088) (8.5607, -55.3417) (8.5001, -55.649) knots 0 0 0 0 1 1 1 1
  spline S229 degree 3 poles (8.5001, -55.649) (8.4815, -55.7375) (8.3838, -55.9889) (8.2813, -56.2077) knots 0 0 0 0 1 1 1 1
  spline S230 degree 3 poles (8.2813, -56.2077) (8.0811, -56.636) (8.0718, -56.664) (7.9182, -57.0457) knots 0 0 0 0 1 1 1 1
  spline S231 degree 3 poles (7.9182, -57.0457) (7.7925, -57.353) (7.4433, -58.0188) (7.2664, -58.2841) knots 0 0 0 0 1 1 1 1
  spline S232 degree 3 poles (7.2664, -58.2841) (7.1966, -58.3912) (7.0383, -58.6613) (6.9126, -58.8894) knots 0 0 0 0 1 1 1 1
  spline S233 degree 3 poles (6.9126, -58.8894) (6.703, -59.2805) (6.3958, -59.746) (6.3539, -59.746) knots 0 0 0 0 1 1 1 1
  spline S234 degree 3 poles (6.3539, -59.746) (6.3446, -59.746) (6.2235, -59.6576) (6.0885, -59.5458) knots 0 0 0 0 1 1 1 1
  spline S235 degree 3 poles (6.0885, -59.5458) (5.7672, -59.2851) (5.3575, -59.1129) (5.2225, -59.1827) knots 0 0 0 0 1 1 1 1
  spline S236 degree 3 poles (5.2225, -59.1827) (5.1108, -59.2432) (5.1387, -59.3596) (5.2784, -59.4015) knots 0 0 0 0 1 1 1 1
  spline S237 degree 3 poles (5.2784, -59.4015) (5.4507, -59.4527) (6.0512, -59.923) (6.1211, -60.0626) knots 0 0 0 0 1 1 1 1
  spline S238 degree 3 poles (6.1211, -60.0626) (6.1583, -60.1325) (6.2701, -60.4211) (6.3678, -60.7005) knots 0 0 0 0 1 1 1 1
  line L24 (6.3678, -60.7005) -> (6.5448, -61.2126)
  line L25 (6.5448, -61.2126) -> (6.5448, -62.0972)
  spline S239 degree 3 poles (6.5448, -62.0972) (6.5448, -62.8421) (6.5308, -63.0237) (6.4563, -63.2378) knots 0 0 0 0 1 1 1 1
  spline S240 degree 3 poles (6.4563, -63.2378) (6.3492, -63.5451) (6.0373, -64.2341) (5.9674, -64.3179) knots 0 0 0 0 1 1 1 1
  spline S241 degree 3 poles (5.9674, -64.3179) (5.9023, -64.3924) (5.6695, -64.709) (5.4739, -64.9884) knots 0 0 0 0 1 1 1 1
  spline S242 degree 3 poles (5.4739, -64.9884) (5.2784, -65.2584) (4.9153, -65.6448) (4.7849, -65.71) knots 0 0 0 0 1 1 1 1
  spline S243 degree 3 poles (4.7849, -65.71) (4.729, -65.7426) (4.5987, -65.8357) (4.4962, -65.9195) knots 0 0 0 0 1 1 1 1
  spline S244 degree 3 poles (4.4962, -65.9195) (4.2029, -66.1569) (3.7606, -66.3944) (3.5139, -66.4549) knots 0 0 0 0 1 1 1 1
  spline S245 degree 3 poles (3.5139, -66.4549) (3.3882, -66.4828) (3.1228, -66.5061) (2.9226, -66.5015) knots 0 0 0 0 1 1 1 1
  spline S246 degree 3 poles (2.9226, -66.5015) (2.5921, -66.5015) (2.5269, -66.4828) (2.2615, -66.3385) knots 0 0 0 0 1 1 1 1
  spline S247 degree 3 poles (2.2615, -66.3385) (1.9961, -66.1849) (1.9589, -66.1476) (1.8052, -65.8357) knots 0 0 0 0 1 1 1 1
  spline S248 degree 3 poles (1.8052, -65.8357) (1.7168, -65.6495) (1.6051, -65.3887) (1.5585, -65.263) knots 0 0 0 0 1 1 1 1
  spline S249 degree 3 poles (1.5585, -65.263) (1.4235, -64.8952) (0.9393, -63.9781) (0.7577, -63.7499) knots 0 0 0 0 1 1 1 1
  spline S250 degree 3 poles (0.7577, -63.7499) (0.6693, -63.6335) (0.5063, -63.4613) (0.4039, -63.3589) knots 0 0 0 0 1 1 1 1
  line L26 (0.4039, -63.3589) -> (0.213, -63.1819)
  line L27 (0.213, -63.1819) -> (-0.1874, -63.2099)
  spline S251 degree 3 poles (-0.1874, -63.2099) (-0.4062, -63.2285) (-0.6576, -63.2611) (-0.7461, -63.2844) knots 0 0 0 0 1 1 1 1
  spline S252 degree 3 poles (-0.7461, -63.2844) (-0.9835, -63.3542) (-1.8774, -63.3402) (-2.2778, -63.2657) knots 0 0 0 0 1 1 1 1
  spline S253 degree 3 poles (-2.2778, -63.2657) (-2.9063, -63.1447) (-3.4464, -63.005) (-3.5907, -62.9305) knots 0 0 0 0 1 1 1 1
  spline S254 degree 3 poles (-3.5907, -62.9305) (-3.6699, -62.8886) (-3.8514, -62.8141) (-3.9911, -62.7676) knots 0 0 0 0 1 1 1 1
  spline S255 degree 3 poles (-3.9911, -62.7676) (-4.1308, -62.721) (-4.3123, -62.6326) (-4.3915, -62.572) knots 0 0 0 0 1 1 1 1
  spline S256 degree 3 poles (-4.3915, -62.572) (-4.4706, -62.5115) (-4.6103, -62.4324) (-4.6988, -62.3998) knots 0 0 0 0 1 1 1 1
  spline S257 degree 3 poles (-4.6988, -62.3998) (-4.7872, -62.3625) (-4.9269, -62.2927) (-5.006, -62.2368) knots 0 0 0 0 1 1 1 1
  spline S258 degree 3 poles (-5.006, -62.2368) (-5.0852, -62.1856) (-5.2388, -62.0925) (-5.3459, -62.0273) knots 0 0 0 0 1 1 1 1
  spline S259 degree 3 poles (-5.3459, -62.0273) (-5.4576, -61.9622) (-5.6439, -61.8364) (-5.7603, -61.748) knots 0 0 0 0 1 1 1 1
  spline S260 degree 3 poles (-5.7603, -61.748) (-5.8813, -61.6549) (-6.1281, -61.4966) (-6.3143, -61.3848) knots 0 0 0 0 1 1 1 1
  spline S261 degree 3 poles (-6.3143, -61.3848) (-6.5564, -61.2452) (-6.7799, -61.045) (-7.1477, -60.6539) knots 0 0 0 0 1 1 1 1
  spline S262 degree 3 poles (-7.1477, -60.6539) (-7.6365, -60.1278) (-7.8181, -60.0114) (-7.8181, -60.2163) knots 0 0 0 0 1 1 1 1
  spline S263 degree 3 poles (-7.8181, -60.2163) (-7.8181, -60.2721) (-7.6132, -60.5189) (-7.2827, -60.8541) knots 0 0 0 0 1 1 1 1
  spline S264 degree 3 poles (-7.2827, -60.8541) (-6.8357, -61.3104) (-6.7612, -61.4081) (-6.8125, -61.464) knots 0 0 0 0 1 1 1 1
  spline S265 degree 3 poles (-6.8125, -61.464) (-6.8497, -61.4966) (-7.1337, -61.5897) (-7.4503, -61.6735) knots 0 0 0 0 1 1 1 1
  spline S266 degree 3 poles (-7.4503, -61.6735) (-7.7622, -61.7526) (-8.0276, -61.8411) (-8.0369, -61.8737) knots 0 0 0 0 1 1 1 1
  spline S267 degree 3 poles (-8.0369, -61.8737) (-8.0788, -61.9994) (-7.427, -61.9947) (-6.9661, -61.8597) knots 0 0 0 0 1 1 1 1
  spline S268 degree 3 poles (-6.9661, -61.8597) (-6.8963, -61.8364) (-6.8869, -61.869) (-6.8869, -62.0925) knots 0 0 0 0 1 1 1 1
  spline S269 degree 3 poles (-6.8869, -62.0925) (-6.8869, -62.2368) (-6.8963, -62.3532) (-6.9056, -62.3532) knots 0 0 0 0 1 1 1 1
  spline S270 degree 3 poles (-6.9056, -62.3532) (-6.9149, -62.3532) (-7.0173, -62.316) (-7.129, -62.2648) knots 0 0 0 0 1 1 1 1
  spline S271 degree 3 poles (-7.129, -62.2648) (-7.3758, -62.1623) (-7.5248, -62.1996) (-7.5667, -62.3858) knots 0 0 0 0 1 1 1 1
  spline S272 degree 3 poles (-7.5667, -62.3858) (-7.6784, -62.884) (-7.6784, -62.884) (-7.7669, -62.7862) knots 0 0 0 0 1 1 1 1
  spline S273 degree 3 poles (-7.7669, -62.7862) (-7.8134, -62.735) (-7.8786, -62.6512) (-7.9065, -62.5953) knots 0 0 0 0 1 1 1 1
  spline S274 degree 3 poles (-7.9065, -62.5953) (-7.9624, -62.4929) (-8.2278, -62.3532) (-8.3675, -62.3532) knots 0 0 0 0 1 1 1 1
  spline S275 degree 3 poles (-8.3675, -62.3532) (-8.4047, -62.3532) (-8.4792, -62.3905) (-8.5258, -62.4324) knots 0 0 0 0 1 1 1 1
  spline S276 degree 3 poles (-8.5258, -62.4324) (-8.6142, -62.5115) (-8.6189, -62.5069) (-8.7073, -62.3998) knots 0 0 0 0 1 1 1 1
  spline S277 degree 3 poles (-8.7073, -62.3998) (-8.9075, -62.1437) (-9.0844, -61.7852) (-9.0612, -61.6921) knots 0 0 0 0 1 1 1 1
  spline S278 degree 3 poles (-9.0612, -61.6921) (-9.0286, -61.5804) (-9.1915, -61.3988) (-9.4476, -61.2545) knots 0 0 0 0 1 1 1 1
  spline S279 degree 3 poles (-9.4476, -61.2545) (-10.1134, -60.882) (-10.7093, -60.2442) (-11.0072, -59.5924) knots 0 0 0 0 1 1 1 1
  spline S280 degree 3 poles (-11.0072, -59.5924) (-11.1935, -59.192) (-11.3192, -58.5262) (-11.2959, -58.1165) knots 0 0 0 0 1 1 1 1
  spline S281 degree 3 poles (-11.2959, -58.1165) (-11.24, -57.2366) (-11.0957, -56.799) (-10.6255, -56.0541) knots 0 0 0 0 1 1 1 1
  line L28 (-10.6255, -56.0541) -> (-10.4998, -55.8585)
  line L29 (-10.4998, -55.8585) -> (-10.3787, -56.2543)
  spline S282 degree 3 poles (-10.3787, -56.2543) (-10.0854, -57.204) (-9.834, -57.6975) (-9.6524, -57.6975) knots 0 0 0 0 1 1 1 1
  spline S283 degree 3 poles (-9.6524, -57.6975) (-9.5128, -57.6975) (-9.5407, -57.5346) (-9.834, -56.7105) knots 0 0 0 0 1 1 1 1
  spline S284 degree 3 poles (-9.834, -56.7105) (-10.1692, -55.7701) (-10.2577, -55.4023) (-10.3322, -54.6667) knots 0 0 0 0 1 1 1 1
  spline S285 degree 3 poles (-10.3322, -54.6667) (-10.388, -54.1173) (-10.402, -52.9347) (-10.3601, -52.5064) knots 0 0 0 0 1 1 1 1
  spline S286 degree 3 poles (-10.3601, -52.5064) (-10.3461, -52.3528) (-10.3089, -51.9524) (-10.281, -51.6218) knots 0 0 0 0 1 1 1 1
  spline S287 degree 3 poles (-10.281, -51.6218) (-10.253, -51.2866) (-10.1785, -50.8071) (-10.1227, -50.551) knots 0 0 0 0 1 1 1 1
  spline S288 degree 3 poles (-10.1227, -50.551) (-9.9923, -50.011) (-9.5779, -48.8284) (-9.4709, -48.712) knots 0 0 0 0 1 1 1 1
  spline S289 degree 3 poles (-9.4709, -48.712) (-9.4336, -48.6701) (-9.401, -48.6096) (-9.401, -48.5817) knots 0 0 0 0 1 1 1 1
  spline S290 degree 3 poles (-9.401, -48.5817) (-9.401, -48.5537) (-9.3731, -48.5025) (-9.3358, -48.4699) knots 0 0 0 0 1 1 1 1
  spline S291 degree 3 poles (-9.3358, -48.4699) (-9.3033, -48.4327) (-9.1915, -48.2418) (-9.0938, -48.0416) knots 0 0 0 0 1 1 1 1
  spline S292 degree 3 poles (-9.0938, -48.0416) (-8.9448, -47.739) (-8.9261, -47.6738) (-8.982, -47.6366) knots 0 0 0 0 1 1 1 1
  spline S293 degree 3 poles (-8.982, -47.6366) (-9.1031, -47.5621) (-9.1869, -47.6133) (-9.2846, -47.8088) knots 0 0 0 0 1 1 1 1
  spline S294 degree 3 poles (-9.2846, -47.8088) (-9.3358, -47.9112) (-9.4197, -48.0556) (-9.4755, -48.1347) knots 0 0 0 0 1 1 1 1
  spline S295 degree 3 poles (-9.4755, -48.1347) (-9.5267, -48.2092) (-9.5966, -48.3396) (-9.6292, -48.4187) knots 0 0 0 0 1 1 1 1
  spline S296 degree 3 poles (-9.6292, -48.4187) (-9.6664, -48.5025) (-9.7083, -48.5723) (-9.7316, -48.5723) knots 0 0 0 0 1 1 1 1
  spline S297 degree 3 poles (-9.7316, -48.5723) (-9.7502, -48.5723) (-9.848, -48.4141) (-9.9411, -48.2232) knots 0 0 0 0 1 1 1 1
  spline S298 degree 3 poles (-9.9411, -48.2232) (-10.0342, -48.0323) (-10.1413, -47.8507) (-10.1785, -47.8228) knots 0 0 0 0 1 1 1 1
  spline S299 degree 3 poles (-10.1785, -47.8228) (-10.2111, -47.7948) (-10.2391, -47.7483) (-10.2391, -47.725) knots 0 0 0 0 1 1 1 1
  spline S300 degree 3 poles (-10.2391, -47.725) (-10.2391, -47.6971) (-10.2949, -47.5993) (-10.3648, -47.5062) knots 0 0 0 0 1 1 1 1
  spline S301 degree 3 poles (-10.3648, -47.5062) (-10.4393, -47.4131) (-10.5277, -47.2641) (-10.5696, -47.1756) knots 0 0 0 0 1 1 1 1
  spline S302 degree 3 poles (-10.5696, -47.1756) (-11.1004, -46.0257) (-11.5799, -45.183) (-11.8267, -44.9549) knots 0 0 0 0 1 1 1 1
  spline S303 degree 3 poles (-11.8267, -44.9549) (-11.8872, -44.9037) (-12.1013, -44.8012) (-12.3015, -44.7314) knots 0 0 0 0 1 1 1 1
  spline S304 degree 3 poles (-12.3015, -44.7314) (-12.4971, -44.6616) (-12.66, -44.5917) (-12.66, -44.5731) knots 0 0 0 0 1 1 1 1
  spline S305 degree 3 poles (-12.66, -44.5731) (-12.66, -44.5591) (-12.5762, -44.4753) (-12.4738, -44.3822) knots 0 0 0 0 1 1 1 1
  spline S306 degree 3 poles (-12.4738, -44.3822) (-12.3248, -44.2519) (-12.2783, -44.1727) (-12.2457, -43.9865) knots 0 0 0 0 1 1 1 1
  spline S307 degree 3 poles (-12.2457, -43.9865) (-12.2084, -43.8003) (-12.2177, -43.7304) (-12.2736, -43.6373) knots 0 0 0 0 1 1 1 1
  spline S308 degree 3 poles (-12.2736, -43.6373) (-12.3807, -43.479) (-12.7485, -43.1159) (-12.9161, -43.0088) knots 0 0 0 0 1 1 1 1
  line L30 (-12.9161, -43.0088) -> (-13.0558, -42.9203)
  line L31 (-13.0558, -42.9203) -> (-12.7764, -42.8598)
  spline S309 degree 3 poles (-12.7764, -42.8598) (-12.6228, -42.8319) (-12.3388, -42.8039) (-12.1432, -42.7993) knots 0 0 0 0 1 1 1 1
  spline S310 degree 3 poles (-12.1432, -42.7993) (-11.7801, -42.7993) (-11.6311, -42.7341) (-11.7056, -42.6084) knots 0 0 0 0 1 1 1 1
  spline S311 degree 3 poles (-11.7056, -42.6084) (-11.7242, -42.5805) (-11.7801, -42.4129) (-11.822, -42.2313) knots 0 0 0 0 1 1 1 1
  line L32 (-11.822, -42.2313) -> (-11.9058, -41.91)
  line L33 (-11.9058, -41.91) -> (-11.808, -41.9426)
  spline S312 degree 3 poles (-11.808, -41.9426) (-11.7522, -41.9613) (-11.6404, -42.0218) (-11.5659, -42.0776) knots 0 0 0 0 1 1 1 1
  spline S313 degree 3 poles (-11.5659, -42.0776) (-11.3471, -42.2406) (-11.0445, -42.3989) (-10.5184, -42.6363) knots 0 0 0 0 1 1 1 1
  spline S314 degree 3 poles (-10.5184, -42.6363) (-10.0156, -42.8645) (-9.4895, -43.1624) (-8.9075, -43.5488) knots 0 0 0 0 1 1 1 1
  spline S315 degree 3 poles (-8.9075, -43.5488) (-8.726, -43.6699) (-8.5304, -43.7816) (-8.4792, -43.8003) knots 0 0 0 0 1 1 1 1
  spline S316 degree 3 poles (-8.4792, -43.8003) (-8.4233, -43.8142) (-8.2185, -43.9446) (-8.0183, -44.0889) knots 0 0 0 0 1 1 1 1
  spline S317 degree 3 poles (-8.0183, -44.0889) (-7.8181, -44.2286) (-7.5481, -44.4008) (-7.413, -44.4614) knots 0 0 0 0 1 1 1 1
  spline S318 degree 3 poles (-7.413, -44.4614) (-7.2734, -44.5265) (-7.1663, -44.6103) (-7.1663, -44.6476) knots 0 0 0 0 1 1 1 1
  spline S319 degree 3 poles (-7.1663, -44.6476) (-7.1663, -44.6895) (-7.2222, -44.8385) (-7.2873, -44.9875) knots 0 0 0 0 1 1 1 1
  spline S320 degree 3 poles (-7.2873, -44.9875) (-7.3525, -45.1364) (-7.3991, -45.304) (-7.3898, -45.3646) knots 0 0 0 0 1 1 1 1
  spline S321 degree 3 poles (-7.3898, -45.3646) (-7.3665, -45.5322) (-7.2268, -45.5275) (-7.0825, -45.3506) knots 0 0 0 0 1 1 1 1
  spline S322 degree 3 poles (-7.0825, -45.3506) (-6.7706, -44.9642) (-5.9558, -44.2239) (-5.6299, -44.0284) knots 0 0 0 0 1 1 1 1
  spline S323 degree 3 poles (-5.6299, -44.0284) (-5.439, -43.912) (-5.1876, -43.7584) (-5.0759, -43.6932) knots 0 0 0 0 1 1 1 1
  spline S324 degree 3 poles (-5.0759, -43.6932) (-4.8245, -43.5395) (-4.7407, -43.4185) (-4.8384, -43.358) knots 0 0 0 0 1 1 1 1
  spline S325 degree 3 poles (-4.8384, -43.358) (-4.9083, -43.3161) (-5.0992, -43.3393) (-5.1876, -43.4045) knots 0 0 0 0 1 1 1 1
  spline S326 degree 3 poles (-5.1876, -43.4045) (-5.2109, -43.4231) (-5.2994, -43.4604) (-5.3785, -43.4837) knots 0 0 0 0 1 1 1 1
  spline S327 degree 3 poles (-5.3785, -43.4837) (-5.6299, -43.5721) (-6.6355, -44.2658) (-6.6774, -44.3869) knots 0 0 0 0 1 1 1 1
  spline S328 degree 3 poles (-6.6774, -44.3869) (-6.6914, -44.4288) (-6.7473, -44.5033) (-6.8031, -44.5498) knots 0 0 0 0 1 1 1 1
  line L34 (-6.8031, -44.5498) -> (-6.9009, -44.6383)
  line L35 (-6.9009, -44.6383) -> (-6.8683, -44.4241)
  spline S329 degree 3 poles (-6.8683, -44.4241) (-6.8311, -44.1774) (-6.8963, -43.1159) (-7.0313, -41.8216) knots 0 0 0 0 1 1 1 1
  spline S330 degree 3 poles (-7.0313, -41.8216) (-7.2128, -40.0431) (-7.2594, -39.247) (-7.3479, -36.7795) knots 0 0 0 0 1 1 1 1
  spline S331 degree 3 poles (-7.3479, -36.7795) (-7.3711, -36.1137) (-7.4037, -35.7459) (-7.4363, -35.7133) knots 0 0 0 0 1 1 1 1
  spline S332 degree 3 poles (-7.4363, -35.7133) (-7.4689, -35.6807) (-7.4922, -35.6202) (-7.4922, -35.5736) knots 0 0 0 0 1 1 1 1
  spline S333 degree 3 poles (-7.4922, -35.5736) (-7.4922, -35.4945) (-7.4875, -35.4898) (-7.3711, -35.5643) knots 0 0 0 0 1 1 1 1
  spline S334 degree 3 poles (-7.3711, -35.5643) (-7.2873, -35.6248) (-7.2687, -35.6528) (-7.3153, -35.6807) knots 0 0 0 0 1 1 1 1
  spline S335 degree 3 poles (-2.8458, -63.4659) (-2.4175, -63.5777) (-1.8076, -63.6568) (-1.4072, -63.6568) knots 0 0 0 0 1 1 1 1
  spline S336 degree 3 poles (-1.4072, -63.6568) (-1.2442, -63.6568) (-1.1139, -63.6661) (-1.1139, -63.6801) knots 0 0 0 0 1 1 1 1
  spline S337 degree 3 poles (-1.1139, -63.6801) (-1.1139, -63.6941) (-1.1558, -63.7872) (-1.207, -63.885) knots 0 0 0 0 1 1 1 1
  spline S338 degree 3 poles (-1.207, -63.885) (-1.2535, -63.9827) (-1.342, -64.1969) (-1.3979, -64.3598) knots 0 0 0 0 1 1 1 1
  spline S339 degree 3 poles (-1.3979, -64.3598) (-1.4537, -64.5228) (-1.5236, -64.6718) (-1.5469, -64.6904) knots 0 0 0 0 1 1 1 1
  spline S340 degree 3 poles (-1.5469, -64.6904) (-1.6912, -64.7789) (-2.464, -64.2574) (-2.897, -63.7825) knots 0 0 0 0 1 1 1 1
  spline S341 degree 3 poles (-2.897, -63.7825) (-3.0646, -63.5963) (-3.2183, -63.4334) (-3.2369, -63.4101) knots 0 0 0 0 1 1 1 1
  spline S342 degree 3 poles (-3.2369, -63.4101) (-3.2881, -63.3589) (-3.2369, -63.3682) (-2.8458, -63.4659) knots 0 0 0 0 1 1 1 1
  spline S343 degree 3 poles (-4.2565, -46.0769) (-4.3403, -46.1374) (-4.3403, -46.1514) (-4.2611, -46.4354) knots 0 0 0 0 1 1 1 1
  line L36 (-4.2611, -46.4354) -> (-4.182, -46.7333)
  line L37 (-4.182, -46.7333) -> (-4.2937, -46.8265)
  spline S344 degree 3 poles (-4.2937, -46.8265) (-4.5312, -47.022) (-4.587, -47.0732) (-4.7081, -47.2175) knots 0 0 0 0 1 1 1 1
  spline S345 degree 3 poles (-4.7081, -47.2175) (-4.9316, -47.4829) (-5.2435, -47.9811) (-5.3645, -48.2744) knots 0 0 0 0 1 1 1 1
  spline S346 degree 3 poles (-5.3645, -48.2744) (-5.5135, -48.6236) (-5.602, -49.2707) (-5.5694, -49.7502) knots 0 0 0 0 1 1 1 1
  spline S347 degree 3 poles (-5.5694, -49.7502) (-5.5368, -50.2112) (-5.3878, -50.5324) (-5.0293, -50.8955) knots 0 0 0 0 1 1 1 1
  spline S348 degree 3 poles (-5.0293, -50.8955) (-4.4381, -51.5008) (-3.8421, -51.7336) (-2.7806, -51.7708) knots 0 0 0 0 1 1 1 1
  spline S349 degree 3 poles (-2.7806, -51.7708) (-2.208, -51.7941) (-2.1381, -51.7894) (-2.1102, -51.7196) knots 0 0 0 0 1 1 1 1
  spline S350 degree 3 poles (-2.1102, -51.7196) (-2.0636, -51.5986) (-2.3104, -50.8955) (-2.627, -50.2251) knots 0 0 0 0 1 1 1 1
  spline S351 degree 3 poles (-2.627, -50.2251) (-2.7434, -49.9877) (-2.911, -49.5128) (-2.9994, -49.1683) knots 0 0 0 0 1 1 1 1
  spline S352 degree 3 poles (-2.9994, -49.1683) (-3.0926, -48.8284) (-3.2508, -48.3396) (-3.3486, -48.0835) knots 0 0 0 0 1 1 1 1
  spline S353 degree 3 poles (-3.3486, -48.0835) (-3.4464, -47.8274) (-3.5488, -47.5248) (-3.5814, -47.4131) knots 0 0 0 0 1 1 1 1
  spline S354 degree 3 poles (-3.5814, -47.4131) (-3.6093, -47.3013) (-3.6559, -47.1756) (-3.6745, -47.1337) knots 0 0 0 0 1 1 1 1
  spline S355 degree 3 poles (-3.6745, -47.1337) (-3.6978, -47.0918) (-3.7816, -46.8591) (-3.8607, -46.6123) knots 0 0 0 0 1 1 1 1
  spline S356 degree 3 poles (-3.8607, -46.6123) (-4.0237, -46.1002) (-4.1168, -45.9745) (-4.2565, -46.0769) knots 0 0 0 0 1 1 1 1